Autodesk Inventor part; units mm, degrees
(part 3 of 3)
  line L455 (50.25, -72.75) -> (50.25, -62.25)
  line L456 (50.25, -62.25) -> (24.75, -62.25)
  line L457 (24.75, -62.25) -> (24.75, -72.75)
  line L458 (24.75, -57.75) -> (50.25, -57.75)
  line L459 (50.25, -57.75) -> (50.25, -47.25)
  line L460 (50.25, -47.25) -> (24.75, -47.25)
  line L461 (24.75, -47.25) -> (24.75, -57.75)
  line L462 (24.75, -42.75) -> (50.25, -42.75)
  line L463 (50.25, -42.75) -> (50.25, -32.25)
  line L464 (50.25, -32.25) -> (24.75, -32.25)
  line L465 (24.75, -32.25) -> (24.75, -42.75)
  line L466 (24.75, -27.75) -> (50.25, -27.75)
  line L467 (50.25, -27.75) -> (50.25, -17.25)
  line L468 (50.25, -17.25) -> (24.75, -17.25)
  line L469 (24.75, -17.25) -> (24.75, -27.75)
  line L470 (24.75, -12.75) -> (50.25, -12.75)
  line L471 (50.25, -12.75) -> (50.25, -2.25)
  line L472 (50.25, -2.25) -> (24.75, -2.25)
  line L473 (24.75, -2.25) -> (24.75, -12.75)
  line L474 (24.75, 2.25) -> (50.25, 2.25)
  line L475 (50.25, 2.25) -> (50.25, 12.75)
  line L476 (50.25, 12.75) -> (24.75, 12.75)
  line L477 (24.75, 12.75) -> (24.75, 2.25)
  line L478 (24.75, 17.25) -> (50.25, 17.25)
  line L479 (50.25, 17.25) -> (50.25, 27.75)
  line L480 (50.25, 27.75) -> (24.75, 27.75)
  line L481 (24.75, 27.75) -> (24.75, 17.25)
  line L482 (24.75, 32.25) -> (50.25, 32.25)
  line L483 (50.25, 32.25) -> (50.25, 42.75)
  line L484 (50.25, 42.75) -> (24.75, 42.75)
  line L485 (24.75, 42.75) -> (24.75, 32.25)
  line L486 (24.75, 47.25) -> (50.25, 47.25)
  line L487 (50.25, 47.25) -> (50.25, 57.75)
  line L488 (50.25, 57.75) -> (24.75, 57.75)
  line L489 (24.75, 57.75) -> (24.75, 47.25)
  line L490 (24.75, 62.25) -> (50.25, 62.25)
  line L491 (50.25, 62.25) -> (50.25, 72.75)
  line L492 (50.25, 72.75) -> (24.75, 72.75)
  line L493 (24.75, 72.75) -> (24.75, 62.25)
  line L494 (24.75, 77.25) -> (50.25, 77.25)
  line L495 (50.25, 77.25) -> (50.25, 87.75)
  line L496 (50.25, 87.75) -> (24.75, 87.75)
  line L497 (24.75, 87.75) -> (24.75, 77.25)
  line L498 (24.75, 92.25) -> (50.25, 92.25)
  line L499 (50.25, 92.25) -> (50.25, 102.75)
  line L500 (50.25, 102.75) -> (24.75, 102.75)
  line L501 (24.75, 102.75) -> (24.75, 92.25)
  line L502 (24.75, 107.25) -> (50.25, 107.25)
  line L503 (50.25, 107.25) -> (50.25, 117.75)
  line L504 (50.25, 117.75) -> (24.75, 117.75)
  line L505 (24.75, 117.75) -> (24.75, 107.25)
  line L506 (9.75, -87.75) -> (20.25, -87.75)
  line L507 (20.25, -87.75) -> (20.25, -69.75)
  line L508 (20.25, -69.75) -> (9.75, -69.75)
  line L509 (9.75, -69.75) -> (9.75, -87.75)
  line L510 (9.75, -47.25) -> (20.25, -47.25)
  line L511 (20.25, -47.25) -> (20.25, -65.25)
  line L512 (20.25, -65.25) -> (9.75, -65.25)
  line L513 (9.75, -65.25) -> (9.75, -47.25)
  line L514 (9.75, -42.75) -> (20.25, -42.75)
  line L515 (20.25, -42.75) -> (20.25, -24.75)
  line L516 (20.25, -24.75) -> (9.75, -24.75)
  line L517 (9.75, -24.75) -> (9.75, -42.75)
  line L518 (9.75, -20.25) -> (20.25, -20.25)
  line L519 (20.25, -20.25) -> (20.25, -9.75)
  line L520 (20.25, -9.75) -> (9.75, -9.75)
  line L521 (9.75, -9.75) -> (9.75, -20.25)
  line L522 (9.75, 12.75) -> (20.25, 12.75)
  line L523 (20.25, 12.75) -> (20.25, -5.25)
  line L524 (20.25, -5.25) -> (9.75, -5.25)
  line L525 (9.75, -5.25) -> (9.75, 12.75)
  line L526 (9.75, 17.25) -> (20.25, 17.25)
  line L527 (20.25, 17.25) -> (20.25, 35.25)
  line L528 (20.25, 35.25) -> (9.75, 35.25)
  line L529 (9.75, 35.25) -> (9.75, 17.25)
  line L530 (9.75, 57.75) -> (20.25, 57.75)
  line L531 (20.25, 57.75) -> (20.25, 39.75)
  line L532 (20.25, 39.75) -> (9.75, 39.75)
  line L533 (9.75, 39.75) -> (9.75, 57.75)
  line L534 (9.75, 62.25) -> (20.25, 62.25)
  line L535 (20.25, 62.25) -> (20.25, 80.25)
  line L536 (20.25, 80.25) -> (9.75, 80.25)
  line L537 (9.75, 80.25) -> (9.75, 62.25)
  line L538 (9.75, 117.75) -> (20.25, 117.75)
  line L539 (20.25, 117.75) -> (20.25, 99.75)
  line L540 (20.25, 99.75) -> (9.75, 99.75)
  line L541 (9.75, 99.75) -> (9.75, 117.75)
  line L542 (9.75, 84.75) -> (20.25, 84.75)
  line L543 (20.25, 84.75) -> (20.25, 95.25)
  line L544 (20.25, 95.25) -> (9.75, 95.25)
  line L545 (9.75, 95.25) -> (9.75, 84.75)
  point P0 (0, 0)
  point P1 (9.75, -64.25)
  point P2 (20.25, -53.75)
  point P3 (20.25, -49.25)
  point P4 (20.25, -8.75)
  point P5 (20.25, -4.25)
  point P6 (20.25, 36.25)
  point P7 (9.75, 40.75)
  point P8 (20.25, 51.25)
  point P9 (20.25, 55.75)
  point P10 (20.25, 96.25)
  point P11 (20.25, 100.75)
  point P12 (35.25, 27.75)
  point P13 (35.25, 17.25)
  point P14 (39.75, 17.25)
  point P15 (39.75, 27.75)
  point P16 (35.25, 42.75)
  point P17 (35.25, 57.75)
  point P18 (35.25, 72.75)
  point P19 (35.25, 92.25)
  point P20 (35.25, -47.25)
  point P21 (35.25, -77.25)
  point P22 (35.25, -32.25)
  point P23 (39.75, -32.25)
  point P24 (35.25, -17.25)
  point P25 (39.75, -17.25)
  point P26 (35.25, -2.25)
  point P27 (39.75, -12.75)
  point P28 (39.75, -2.25)
  point P29 (35.25, 12.75)
  point P30 (35.25, 2.25)
  point P31 (39.75, 2.25)
  point P32 (39.75, 12.75)
  point P33 (9.75, 99.75)
  point P34 (20.25, 99.75)
  point P35 (20.25, 102.75)
  point P36 (9.75, 107.25)
  point P37 (9.75, 102.75)
  point P38 (9.75, 95.25)
  point P39 (9.75, 92.25)
  point P40 (9.75, 87.75)
  point P41 (20.25, 92.25)
  point P42 (9.75, 80.25)
  point P43 (9.75, 77.25)
  point P44 (9.75, 72.75)
  point P45 (20.25, 72.75)
  point P46 (9.75, 39.75)
  point P47 (20.25, 42.75)
  point P48 (9.75, 47.25)
  point P49 (9.75, 42.75)
  point P50 (20.25, 35.25)
  point P51 (9.75, 35.25)
  point P52 (9.75, 32.25)
  point P53 (9.75, 27.75)
  point P54 (20.25, 27.75)
  point P55 (20.25, 32.25)
  point P56 (9.75, -5.25)
  point P57 (20.25, -5.25)
  point P58 (20.25, -2.25)
  point P59 (20.25, 2.25)
  point P60 (9.75, 2.25)
  point P61 (9.75, -2.25)
  point P62 (9.75, -9.75)
  point P63 (9.75, -12.75)
  point P64 (9.75, -17.25)
  point P65 (20.25, -12.75)
  point P66 (9.75, -24.75)
  point P67 (9.75, -27.75)
  point P68 (9.75, -32.25)
  point P69 (20.25, -27.75)
  point P70 (9.75, -65.25)
  point P71 (20.25, -57.75)
  point P72 (9.75, -57.75)
  point P73 (9.75, -62.25)
  point P74 (9.75, -69.75)
  point P75 (9.75, -72.75)
  point P76 (9.75, -77.25)
  point P77 (20.25, -77.25)
  dimension "d223" = 0.25
  dimension "d224" = 10.5
  dimension "d225" = 10.5
  dimension "d226" = 0.25
  dimension "d229" = 15
  dimension "d232" = 15
  dimension "d283" = 10.5
  dimension "d284" = 18
  dimension "d285" = 18
  dimension "d286" = 18
  dimension "d287" = 10.5
  dimension "d288" = 4.5
  dimension "d289" = 18
  dimension "d290" = 18
  dimension "d291" = 18
  dimension "d292" = 18
  dimension "d293" = 18
  dimension "d294" = 10.5
  dimension "d295" = 4.5
  constraints: 1088 end point, 50 parallel, 26 horizontal, 25 perpendicular, 21 point on line, 2 collinear, 1 vertical, 886 other
  measures "d223" distance between parallel lines of L4 L0
  measures "d224" distance of L0.start L0.end
  measures "d225" distance of L0.end L1.end
  measures "d226" distance between parallel lines of L5 L3
  measures "d229" distance of L0.start L6.start
  measures "d232" distance of L0.start L66.start
  measures "d283" distance of L508.end L507.end
  measures "d284" distance of L507.end L506.end
  measures "d285" distance of L510.end L511.end
  measures "d286" distance of L514.end L515.end
  measures "d287" distance of L518.end L519.end
  measures "d288" distance between parallel lines of L516 L518
  measures "d289" distance of L522.end L523.end
  measures "d290" distance of L526.end L527.end
  measures "d291" distance of L530.end L531.end
  measures "d292" distance of L534.end L535.end
  measures "d293" distance of L538.end L539.end
  measures "d294" distance of L542.end L543.end
  measures "d295" distance between parallel lines of L536 L542
extrude "Extrusion8" add sketch "Sketch21" along normal blind 1 contours L0 L1 L2 L3 | L6 L7 L8 L9 | L66 L67 L68 L69 | L70 L71 L72 L73 | L130 L131 L132 L133 | L134 L135 L136 L137 | L162 L163 L164 L165 | L166 L167 L168 L169 | L170 L171 L172 L173 | L174 L175 L176 L177 | L178 L179 L180 L181 | L182 L183 L184 L185 | L186 L187 L188 L189 | L190 L191 L192 L193 | L194 L195 L196 L197 | L198 L199 L200 L201 | L226 L227 L228 L229 | L230 L231 L232 L233 | L234 L235 L236 L237 | L238 L239 L240 L241 | L242 L243 L244 L245 | L246 L247 L248 L249 | L250 L251 L252 L253 | L254 L255 L256 L257 | L258 L259 L260 L261 | L262 L263 L264 L265 | L266 L267 L268 L269 | L268 L509 L270 L507 | L270 L271 L508 L273 | L512 L271 L272 L273 | L272 L513 L274 L511 | L274 L275 L276 L277 | L278 L279 L280 L281 | L280 L517 L282 L515 | L282 L283 L516 L285 | L518 L283 L284 L285 | L284 L521 L286 L519 | L286 L287 L520 L289 | L524 L287 L288 L289 | L288 L525 L290 L523 | L290 L291 L292 L293 | L294 L295 L296 L297 | L296 L529 L298 L527 | L298 L299 L528 L301 | L532 L299 L300 L301 | L300 L533 L302 L531 | L302 L303 L304 L305 | L306 L307 L308 L309 | L308 L537 L310 L535 | L310 L311 L536 L313 | L542 L311 L312 L313 | L312 L545 L314 L543 | L314 L315 L544 L317 | L540 L315 L316 L317 | L316 L541 L318 L539 | L318 L319 L320 L321 | L322 L323 L324 L325 | L326 L327 L328 L329 | L330 L331 L332 L333 | L333 L452 L395 L450 | L395 L396 L397 L394 | L334 L335 L336 L337 | L337 L456 L399 L454 | L399 L400 L401 L398 | L338 L339 L340 L341 | L341 L460 L403 L458 | L403 L404 L405 L402 | L342 L343 L344 L345 | L345 L464 L407 L462 | L407 L408 L409 L406 | L346 L347 L348 L349 | L349 L468 L411 L466 | L411 L412 L413 L410 | L350 L351 L352 L353 | L353 L472 L415 L470 | L415 L416 L417 L414 | L354 L355 L356 L357 | L357 L476 L419 L474 | L419 L420 L421 L418 | L358 L359 L360 L361 | L361 L480 L423 L478 | L423 L424 L425 L422 | L362 L363 L364 L365 | L365 L484 L427 L482 | L427 L428 L429 L426 | L366 L367 L368 L369 | L369 L488 L431 L486 | L431 L432 L433 L430 | L370 L371 L372 L373 | L373 L492 L435 L490 | L435 L436 L437 L434 | L374 L375 L376 L377 | L377 L496 L439 L494 | L439 L440 L441 L438 | L378 L379 L380 L381 | L381 L500 L443 L498 | L443 L444 L445 L442 | L382 L383 L384 L385 | L385 L504 L447 L502 | L447 L448 L449 L446 | L386 L387 L388 L389 | L390 L391 L392 L393
sketch "Sketch23" plane through (0, 4, 0) normal (0, 1, 0) x (1, 0, 0)
  circle A0 centre (-61, -129) radius 10.25
  line L0 (-60.5, 128.5) -> (-60.5, -128.5) projected
  line L1 (-60.5, -128.5) -> (60.5, -128.5) projected
  circle A1 centre (61, 129) radius 10.25
  circle A2 centre (61, -129) radius 10.25
  line L2 (60.5, -128.5) -> (60.5, 128.5) projected
  line L3 (60.5, 128.5) -> (-60.5, 128.5) projected
  circle A3 centre (-61, 129) radius 10.25
  circle A4 centre (-61, 0) radius 7.75
  circle A5 centre (61, 0) radius 7.75
  point P0 (0, 0)
  point P1 (-50.7622, -128.5)
  point P2 (-60.5, -118.7622)
  dimension "d338" = 20.5
  dimension "d339" = 0.5
  dimension "d340" = 0.5
  dimension "d341" = 20.5
  dimension "d342" = 0.5
  dimension "d343" = 0.5
  dimension "d344" = 20.5
  dimension "d345" = 0.5
  dimension "d346" = 0.5
  dimension "d347" = 0.5
  dimension "d348" = 0.5
  dimension "d349" = 20.5
  dimension "d350" = 15.5
  dimension "d351" = 0.5
  dimension "d352" = 128.5
  dimension "d353" = 15.5
  dimension "d354" = 0.5
  dimension "d355" = 128.5
  constraints: 6 centre point
  measures "d338" diameter of A0
  measures "d339" distance from line of L0 A0.centre
  measures "d340" distance from line of A0.centre L1
  measures "d341" diameter of A2
  measures "d342" distance from line of L2 A2.centre
  measures "d343" distance from line of L1 A2.centre
  measures "d344" diameter of A1
  measures "d345" distance from line of L3 A1.centre
  measures "d346" distance from line of L2 A1.centre
  measures "d347" distance from line of L0 A3.centre
  measures "d348" distance from line of L3 A3.centre
  measures "d349" diameter of A3
  measures "d350" diameter of A4
  measures "d351" distance from line of L0 A4.centre
  measures "d352" distance from line of L3 A4.centre
  measures "d353" diameter of A5
  measures "d354" distance from line of L2 A5.centre
  measures "d355" distance from line of L1 A5.centre
extrude "Extrusion9" cut sketch "Sketch23" against normal through all contours L1 L0 A0 | A2 L2 L1 | L1 L2 A2 | A4 L0 | L0 A4 | A5 L2 | L2 A5 | A3 L3 L0 | L0 L3 A3 | L2 L3 A1 | A1 L3 L2 picked at (-54.151, -127.6755)
body "Solid1"
